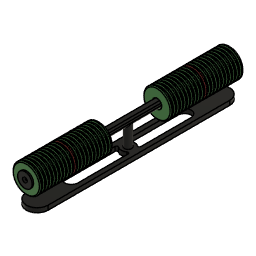
Ping Pong Scorer (Autodesk Fusion 360 design; units mm, degrees)
Autodesk Fusion 360 part; units mm, degrees
note: some values were not read from the file. Chosen so that the rebuilt part matches the saved one: which bodies a step acts on; which face or edge a step refers to; which pieces of a blend or face edit are solid. Set by a fixed rule: the direction of a hole.
sketch "Sketch1" plane through (0, 0, 0) normal (0, 0, 1) x (1, 0, 0)
  line L0 (0, 0) -> (13, 0)
  line L1 (13, 0) -> (13, 36)
  line L2 (13, 36) -> (0, 36)
  line L3 (0, 36) -> (0, 0)
  dimension "d1" = 13
  dimension "d2" = 36
  constraint coincident L0.start L3.end
  constraint horizontal L0
  constraint perpendicular L0 L1
  constraint perpendicular L1 L2
  constraint perpendicular L0 L3
  measures "d1" distance of L0.start L0.end
  measures "d2" distance of L0.end L1.end
extrude "Extrude1" add sketch "Sketch1" along normal blind 3 makes body 1
copy_body "Body->Comp1" bodies 1 removing the originals makes body 2 in component "Magnet"
sketch "Sketch2" plane through (0, 0, 0) normal (0, 0, 1) x (1, 0, 0)
  line L0 (0, 0) -> (13, 0)
  line L1 (6.5, 0) -> (21.5, 0) construction
  line L2 (6.5, 0) -> (-8.5, 0) construction
  line L3 (21.5, 0) -> (21.5, -10)
  line L4 (21.5, -10) -> (-8.5, -10)
  line L5 (-8.5, -10) -> (-8.5, 0)
  line L6 (-8.5, 0) -> (-8.5, 130)
  line L7 (0, 36) -> (0, 0)
  line L8 (13, 36) -> (0, 36)
  line L9 (13, 0) -> (13, 36)
  line L10 (-1, -1) -> (14, -1)
  line L11 (14, -1) -> (14, 37)
  line L12 (14, 37) -> (-1, 37)
  line L13 (-1, 37) -> (-1, -1)
  line L14 (21.5, 0) -> (21.5, 130)
  line L15 (21.5, 130) -> (-8.5, 130) construction
  line L16 (13, 224) -> (0, 224)
  line L17 (21.5, 260) -> (21.5, 270)
  line L18 (0, 260) -> (13, 260)
  line L19 (6.5, 260) -> (21.5, 260) construction
  line L20 (-1, 223) -> (-1, 261)
  line L21 (-8.5, 270) -> (-8.5, 260)
  line L22 (13, 260) -> (13, 224)
  line L23 (-1, 261) -> (14, 261)
  line L24 (6.5, 260) -> (-8.5, 260) construction
  line L25 (14, 223) -> (-1, 223)
  line L26 (0, 224) -> (0, 260)
  line L27 (21.5, 270) -> (-8.5, 270)
  line L28 (14, 261) -> (14, 223)
  line L29 (-8.5, 260) -> (-8.5, 130)
  line L30 (21.5, 260) -> (21.5, 130)
  circle A0 centre (6.5, 130) radius 5
  point P0 (0, 260)
  dimension "d5" = 15
  dimension "d6" = 15
  dimension "d7" = 10
  dimension "d8" = 130
  dimension "d9" = 1
  dimension "d10" = 10
  constraint midpoint L0 L1.start
  constraint parallel L0 L1
  constraint parallel L0 L2
  constraint perpendicular L1 L3
  constraint perpendicular L3 L4
  constraint perpendicular L2 L5
  constraint perpendicular L2 L6
  constraint perpendicular L1 L14
  constraint perpendicular L6 L15
  constraint symmetric L0.start L15 L18.start
  constraint symmetric L0.start L15 P0
  constraint symmetric L0.end L15 L18.end
  constraint symmetric L1.start L15 L19.start
  constraint symmetric L1.end L15 L17.start
  constraint symmetric L2.end L15 L21.end
  constraint symmetric L3.end L15 L17.end
  constraint symmetric L4.end L15 L21.start
  constraint symmetric L6.end L15 L29.end
  constraint symmetric L7.start L15 L16.end
  constraint symmetric L8.start L15 L16.start
  constraint symmetric L10.start L15 L20.end
  constraint symmetric L10.end L15 L23.end
  constraint symmetric L11.end L15 L25.start
  constraint symmetric L12.end L15 L20.start
  constraint symmetric L14.end L15 L30.end
  constraint midpoint L15 A0.centre
  measures "d5" distance of L1.start L1.end
  measures "d6" distance of L1.start L2.end
  measures "d7" distance of L1.end L3.end
  measures "d8" distance of L2.end L6.end
  measures "d10" diameter of A0
extrude "Extrude2" add sketch "Sketch2" along normal blind 6 separate body contours L3 L4 L5 L6 L14 L17 L21 L27 L29 L30 | A0 makes body 3
extrude "Extrude3" add sketch "Sketch2" along normal blind 3.5 from surface at 2.5 contours L0 L7 L8 L9 | L10 L11 L12 L13 | L16 L18 L22 L26 | L20 L23 L25 L28 bodies 3
extrude "Extrude4" add sketch "Sketch2" along normal blind 36 from surface at 6 separate body contours A0 makes body 4
ref_plane "WorkPlane1" through (6.5, 130, 3) normal (0, -1, 0) x (1, 0, 0)
sketch "Sketch3" plane through (0, 130, 0) normal (0, -1, 0) x (-1, 0, 0)
  line L0 (-11.5, -42) -> (-1.5, -42)
  line L1 (-6.5, -42) -> (-6.5, -37) construction
  circle A0 centre (-6.5, -37) radius 5
  line L2 (-11.5, -42) -> (-11.5, -37)
  line L3 (-1.5, -42) -> (-1.5, -37)
  dimension "d19" = 5
  dimension "d20" = 10
  constraint midpoint L0 L1.start
  constraint perpendicular L0 L1
  constraint coincident L1.end A0.centre
  constraint coincident L0.start L2.start
  constraint coincident A0 L2.end
  constraint tangent A0 L2
  constraint coincident L0.end L3.start
  constraint coincident A0 L3.end
  constraint tangent A0 L3
  measures "d19" distance of L1.start L1.end
  measures "d20" diameter of A0
extrude "Extrude5" add sketch "Sketch3" along normal mid plane 280 bodies 3 4
sketch "Sketch4" plane through (0, -10, 0) normal (0, -1, 0) x (1, 0, 0)
  line L0 (11.5, 42) -> (1.5, 42)
  line L1 (1.5, 42) -> (1.5, 37)
  arc A0 (1.5, 37) -> (11.5, 37) centre (6.5, 37) ccw
  line L2 (11.5, 37) -> (11.5, 42)
  arc A1 (1.5, 37) -> (11.5, 37) centre (6.5, 37) ccw
  circle A2 centre (6.5, 37) radius 10
  dimension "d26" = 20
  constraint concentric A1 A2
  measures "d26" diameter of A2
extrude "Extrude6" add sketch "Sketch4" along normal blind 2 separate body contours L0 L1 A0 L2 A1 | A2 makes body 6
copy_body "CopyPasteBodies2" bodies 6 makes body 7
move_body "Move2" bodies 7 to x (1, 0, 0) y (0, 1, 0) z (0, 0, 1) at (0, 282, 0)
hole "Hole1" at (6.5, -12, 37) direction (0, 1, 0) diameter 2.5 depth 40 tip angle 118 countersink diameter 6.5 countersink angle 90 bodies 6 4
hole "Hole2" at (6.5, 272, 37) direction (0, -1, 0) diameter 2.5 depth 40 tip angle 118 countersink diameter 6.5 countersink angle 90 bodies 4 7
hole "Hole3" at (6.5, 130, 0) direction (0, 0, 1) diameter 2.5 depth 40 tip angle 118 countersink diameter 6.5 countersink angle 90 bodies 3 4
copy_body "Body->Comp2" bodies 4 removing the originals makes body 8 in component "Holder"
sketch "Sketch5" plane through (0, 0, 6) normal (0, 0, 1) x (-1, 0, 0)
  circle A0 centre (-6.5, -130) radius 1.25
  line L0 (-21.5, -270) -> (8.5, -270)
  line L1 (8.5, -270) -> (8.5, 10)
  line L2 (8.5, 10) -> (-21.5, 10)
  line L3 (-21.5, 10) -> (-21.5, -270)
  line L4 (2.5, -264) -> (2.5, 4)
  line L5 (2.5, 4) -> (-15.5, 4)
  line L6 (-15.5, 4) -> (-15.5, -264)
  line L7 (-15.5, -264) -> (2.5, -264)
  circle A1 centre (-6.5, -130) radius 9.25
  line L8 (1, 1) -> (1, -37)
  line L9 (1, -37) -> (-14, -37)
  line L10 (-14, -37) -> (-14, 1)
  line L11 (-14, 1) -> (1, 1)
  line L12 (1, -261) -> (-14, -261)
  line L13 (-14, -261) -> (-14, -223)
  line L14 (1, -223) -> (1, -261)
  line L15 (-14, -223) -> (1, -223)
  line L16 (7, -267) -> (-20, -267)
  line L17 (-20, -267) -> (-20, -217)
  line L18 (-20, -217) -> (7, -217)
  line L19 (7, -217) -> (7, -267)
  line L20 (-20, 7) -> (7, 7)
  line L21 (7, 7) -> (7, -43)
  line L22 (7, -43) -> (-20, -43)
  line L23 (-20, -43) -> (-20, 7)
  line L24 (2.5, -43) -> (2.5, -52) construction
  line L25 (-15.5, -43) -> (-15.5, -52) construction
  arc A2 (2.5, -52) -> (-6.5, -43) centre (-6.5, -52) ccw
  arc A3 (-6.5, -43) -> (-15.5, -52) centre (-6.5, -52) ccw
  line L26 (-15.5, -130) -> (2.5, -130) construction
  arc A4 (-6.5, -217) -> (2.5, -208) centre (-6.5, -208) ccw
  arc A5 (-15.5, -208) -> (-6.5, -217) centre (-6.5, -208) ccw
  point P0 (-6.5, -139.25)
  point P1 (-6.5, -120.75)
  point P2 (-6.5, -43)
  dimension "d43" = -6
  dimension "d44" = 8
  dimension "d45" = -6
  dimension "d46" = -6
  dimension "d47" = 9
  dimension "d48" = 9
  constraint coincident A1 P0
  constraint coincident A1 P1
  constraint midpoint L22 P2
  constraint coincident L4 L24.start
  constraint coincident L22 L24.start
  constraint perpendicular L22 L24
  constraint coincident L22 L25.start
  constraint coincident L6 L25.start
  constraint perpendicular L22 L25
  constraint tangent L4 A2
  constraint coincident P2 A2.end
  constraint tangent L25 A3
  constraint midpoint L6 L26.start
  constraint midpoint L4 L26.end
  constraint symmetric L24.end L26 A4.end
  constraint symmetric L25.end L26 A5.start
  constraint symmetric P2 L26 A4.start
  constraint symmetric A2 L26 A4
  constraint symmetric A3 L26 A5
  measures "d47" distance of L24.start L24.end
  measures "d48" distance of L25.start L25.end
extrude "Extrude7" cut sketch "Sketch5" against normal blind 6 contours L4 L6 A1 A4 A5 | L4 L6 A1 A2 A3 bodies 3
fillet "Fillet1" radius 2 4 edges at (-2.5, 127.864, 3) (15.5, 127.864, 3) (15.5, 132.136, 3) (-2.5, 132.136, 3) on bodies 3
fillet "Fillet1" radius 15 4 edges at (21.5, -10, 3) (-8.5, -10, 3) (21.5, 270, 3) (-8.5, 270, 3) on bodies 3
fillet "Fillet1'" radius 2 2 edges at (11.5, 130, 42) (1.5, 130, 42) on bodies 8 in component "Holder"
sketch "Sketch6" plane through (0, -10, 0) normal (0, 1, 0) x (-1, 0, 0)
  circle A0 centre (-6.5, 37) radius 1.25
  circle A1 centre (-6.5, 37) radius 10
  circle A2 centre (-6.5, 37) radius 20
  circle A3 centre (-6.5, 37) radius 6.5
  dimension "d57" = 40
  dimension "d63" = 13
  constraint concentric A0 A2
  constraint concentric A2 A3
  measures "d57" diameter of A2
  measures "d63" diameter of A3
extrude "Extrude8" add sketch "Sketch6" along normal blind 4 separate body contours A1 | A2 makes body 9
chamfer "Chamfer1" distance 2 angle 45 2 edges at (25.1465, -6, 29.7677) (25.1465, -10, 29.7677) on bodies 9
fillet "Fillet2" radius 1 2 edges at (26.5, -8.0004, 37) (26.5, -7.9996, 37) on bodies 9
pattern_linear "R-Pattern1" count 21 spacing 4.8 along (0, 1, 0) of bodies 9 makes body 10 at (-7.5757, -5.2, 35.7828) makes body 11 at (-7.5757, -0.4, 35.7828) makes body 12 at (-7.5757, 4.4, 35.7828) makes body 13 at (-7.5757, 9.2, 35.7828) makes body 14 at (-7.5757, 14, 35.7828) makes body 15 at (-7.5757, 18.8, 35.7828) makes body 16 at (-7.5757, 23.6, 35.7828) makes body 17 at (-7.5757, 28.4, 35.7828) makes body 18 at (-7.5757, 33.2, 35.7828) makes body 19 at (-7.5757, 38, 35.7828) makes body 20 at (-7.5757, 42.8, 35.7828) makes body 21 at (-7.5757, 47.6, 35.7828) makes body 22 at (-7.5757, 52.4, 35.7828) makes body 23 at (-7.5757, 57.2, 35.7828) makes body 24 at (-7.5757, 62, 35.7828) makes body 25 at (-7.5757, 66.8, 35.7828) makes body 26 at (-7.5757, 71.6, 35.7828) makes body 27 at (-7.5757, 76.4, 35.7828) makes body 28 at (-7.5757, 81.2, 35.7828) makes body 29 at (-7.5757, 86, 35.7828)
mirror "Mirror1" about plane through (6.5, 130, 3) normal (0, -1, 0) of bodies 29 14 9 11 10 12 13 27 26 25 24 28 22 23 17 18 16 19 21 15 20 makes body 30 at (-7.5757, 270, 35.7828) makes body 31 at (-7.5757, 265.2, 35.7828) makes body 32 at (-7.5757, 260.4, 35.7828) makes body 33 at (-7.5757, 255.6, 35.7828) makes body 34 at (-7.5757, 250.8, 35.7828) makes body 35 at (-7.5757, 246, 35.7828) makes body 36 at (-7.5757, 241.2, 35.7828) makes body 37 at (-7.5757, 236.4, 35.7828) makes body 38 at (-7.5757, 231.6, 35.7828) makes body 39 at (-7.5757, 226.8, 35.7828) makes body 40 at (-7.5757, 222, 35.7828) makes body 41 at (-7.5757, 217.2, 35.7828) makes body 42 at (-7.5757, 212.4, 35.7828) makes body 43 at (-7.5757, 207.6, 35.7828) makes body 44 at (-7.5757, 202.8, 35.7828) makes body 45 at (-7.5757, 198, 35.7828) makes body 46 at (-7.5757, 193.2, 35.7828) makes body 47 at (-7.5757, 188.4, 35.7828) makes body 48 at (-7.5757, 183.6, 35.7828) makes body 49 at (-7.5757, 178.8, 35.7828) makes body 50 at (-7.5757, 174, 35.7828)
component "Magnet" placed x (1, 0, 0) y (0, 1, 0) z (0, 0, 1) at (0, 0, -0.5)
component "Holder" placed x (1, 0, 0) y (0, 1, 0) z (0, 0, 1) at (0, 0, 0)
component "Magnet" placed x (1, 0, 0) y (0, 1, 0) z (0, 0, 1) at (0, 224, -0.5)
equation "d14 = 6 mm - 2.5 mm"
named bodies: "Magnet"
